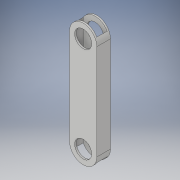
# Autodesk Inventor part: WristBarr.ver1-1111-2020
Saved by Autodesk Inventor 2018 (Build 220112000, 112)
## iProperties
Created: 2020-01-13
Part Number: WristBarr.ver1-1111-2020
Material: Generic
Document SubType Name: Modeling
Designer: JMHal
Density: 1 g/cm^3
Appearance: Default
Author: JMHal
Autodesk Inventor part; units mm, degrees
ref_plane "YZ Plane" through (0, 0, 0) normal (1, 0, 0) x (0, 1, 0)
ref_plane "XZ Plane" through (0, 0, 0) normal (0, 1, 0) x (-1, 0, 0)
ref_plane "XY Plane" through (0, 0, 0) normal (0, 0, 1) x (1, 0, 0)
sketch "Sketch1" plane through (0, 0, 0) normal (0, 1, 0) x (-1, 0, 0)
  line L0 (0, 0) -> (50.8, 0)
  line L1 (50.8, 0) -> (50.8, -25.4)
  line L2 (50.8, -25.4) -> (0, -25.4)
  line L3 (0, -25.4) -> (0, 0)
  line L4 (47.625, -22.225) -> (47.625, -3.175)
  line L5 (47.625, -3.175) -> (3.175, -3.175)
  line L6 (3.175, -3.175) -> (3.175, -22.225)
  line L7 (3.175, -22.225) -> (47.625, -22.225)
  dimension "d0" = 50.8
  dimension "d1" = 25.4
  dimension "d2" = 3.175
  constraints: 16 end point, 4 parallel, 2 perpendicular, 1 horizontal, 3 other
  measures "d0" distance of L1.end L2.end
  measures "d1" distance of L0.end L1.end
  measures "d2" distance between parallel lines of L1 L4
extrude "Extrusion1" add sketch "Sketch1" along normal blind 228.6
sketch "Sketch2" plane through (0, 0, -25.4) normal (0, 0, -1) x (-1, 0, 0)
  line L0 (50.8, 0) -> (0, 0) projected
  line L1 (50.8, 0) -> (50.8, 228.6) projected
  line L2 (0, 228.6) -> (50.8, 228.6) projected
  line L3 (0, 0) -> (0, 228.6) projected
  circle A0 centre (25.4, 203.2) radius 15.875
  circle A1 centre (25.4, 25.4) radius 15.875
  dimension "d5" = 25.4
  dimension "d6" = 25.4
  dimension "d7" = 31.75
  dimension "d8" = 25.4
  dimension "d9" = 25.4
  dimension "d10" = 31.75
  constraints: 2 centre point, 2 coincident
  measures "d5" distance from line of L1 point (25.4, 203.2)
  measures "d6" distance from line of L2 point (25.4, 203.2)
  measures "d7" diameter of A0
  measures "d8" distance from line of L1 point (25.4, 25.4)
  measures "d9" distance from line of L0 point (25.4, 25.4)
  measures "d10" diameter of A1
extrude "Extrusion2" cut sketch "Sketch2" against normal through all contours A0 | A1
fillet "Fillet1" radius 25.4 4 edges at (-50.8, 228.6, -12.7) (0, 228.6, -12.7) (-50.8, 0, -12.7) (0, 0, -12.7)
body "Solid1"
